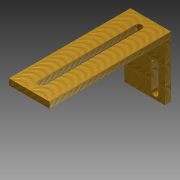
# Autodesk Inventor part: 13_0204_065
Saved by Autodesk Inventor 2012 SP1 (Build 160190100, 190)
## iProperties
Created: 2013-04-30
Part Number: 13_0204_065
Material: Default
Document SubType Name: Modeling
Designer: vogel
Density: 1 g/cm^3
Author: vogel
Autodesk Inventor part; units mm, degrees
ref_plane "YZ Plane" through (0, 0, 0) normal (1, 0, 0) x (0, 1, 0)
ref_plane "XZ Plane" through (0, 0, 0) normal (0, 1, 0) x (-1, 0, 0)
ref_plane "XY Plane" through (0, 0, 0) normal (0, 0, 1) x (1, 0, 0)
sketch "Skizze1" plane through (0, 0, 0) normal (0, 0, 1) x (1, 0, 0)
  line L0 (-10, 30) -> (10, 30)
  line L1 (10, 30) -> (10, -30)
  line L2 (10, -30) -> (-10, -30)
  line L3 (-10, -30) -> (-10, 30)
  line L4 (-14, 0) -> (14, 0) projected
  line L5 (0, -42) -> (0, 42) projected
  line L6 (1.7, 24) -> (1.7, -24)
  line L7 (-1.7, -24) -> (-1.7, 24)
  arc A0 (1.7, 24) -> (-1.7, 24) centre (0, 24) ccw
  arc A1 (-1.7, -24) -> (1.7, -24) centre (0, -24) ccw
  point P0 (0, 0)
  dimension "d0" = 20
  dimension "d1" = 3.4
  dimension "d2" = 60
  dimension "d3" = 48
  constraints: 12 end point, 4 point on circle, 4 tangent, 3 parallel, 2 centre point, 1 horizontal, 1 perpendicular, 1 symmetric about line, 3 other
  measures "d0" distance of L1.end L2.end
  measures "d1" distance between parallel lines of L7 L6
  measures "d2" distance between parallel lines of L2 L0
  measures "d3" distance of A1.centre A0.centre
extrude "Extrusion1" add sketch "Skizze1" along normal blind 3 contours L0 L5 A0 L7 L4 L3 | L0 L1 L4 L6 A0 L5 | L4 L7 A1 L5 L2 L3 | L1 L2 L5 A1 L6 L4
sketch "Skizze2" plane through (10, -30, 0) normal (1, 0, 0) x (0, 0, -1)
  line L0 (-3, 60) -> (-3, 0) projected
  line L1 (0, 60) -> (27, 60)
  line L2 (27, 60) -> (27, 57)
  line L3 (27, 57) -> (0, 57)
  line L4 (0, 57) -> (0, 60)
  point P0 (0, 30)
  dimension "d6" = 3
  dimension "d7" = 30
  constraints: 8 end point, 2 parallel, 1 horizontal, 1 perpendicular
  measures "d6" distance between parallel lines of L3 L1
  measures "d7" distance between parallel lines of L2 L0
extrude "Extrusion2" add sketch "Skizze2" against normal up to surface (20 mm away)
sketch "Skizze3" plane through (-10, 30, 3) normal (0, 1, 0) x (1, 0, 0)
  line L0 (0, 0) -> (20, 0) projected
  line L1 (20, 30) -> (0, 30) projected
  line L2 (10, 30) -> (10, 0)
  line L3 (13, 30) -> (17, 30)
  line L4 (17, 30) -> (17, 18.0571)
  line L5 (17, 18.0571) -> (13, 18.0571)
  line L6 (13, 18.0571) -> (13, 30)
  line L7 (16.7, 27) -> (16.7, 15)
  line L8 (13.3, 15) -> (13.3, 27)
  arc A0 (16.7, 27) -> (13.3, 27) centre (15, 27) ccw
  arc A1 (13.3, 15) -> (16.7, 15) centre (15, 15) ccw
  line L9 (15, 27) -> (15, 15)
  point P0 (10, 3)
  dimension "d10" = 3
  dimension "d11" = 4
  dimension "d12" = 2
  dimension "d13" = 3.4
  dimension "d14" = 3
  dimension "d15" = 12
  constraints: 16 end point, 4 parallel, 4 point on circle, 4 tangent, 2 centre point, 2 midpoint, 1 horizontal, 1 perpendicular, 1 point on line
  measures "d10" distance between parallel lines of L2 L6
  measures "d11" distance between parallel lines of L6 L4
  measures "d12" distance between parallel lines of L6 L9
  measures "d13" distance between parallel lines of L7 L8
  measures "d14" distance from line of L1 L9.start
  measures "d15" distance of L9.end L9.start
extrude "Extrusion3" cut sketch "Skizze3" against normal blind 3 contours L7 A1 L8 L5 | L5 L8 A0 L7
